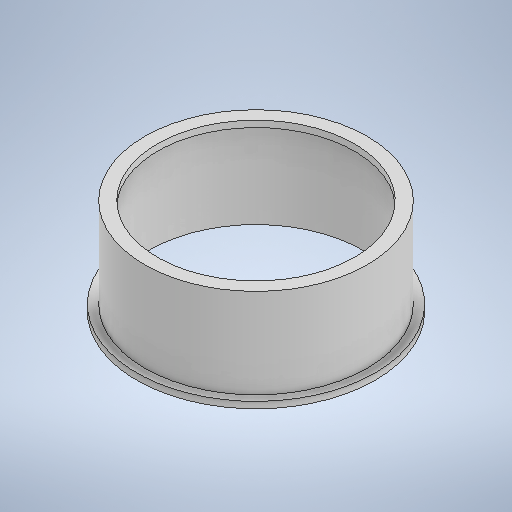
# Autodesk Inventor part: Cylinder Replacement- 10
Saved by Autodesk Inventor 2025.2 (Build 292293000, 293)
## iProperties
Created: 2024-04-11
Part Number: Cylinder Replacement- 10
Material: Generic
Document SubType Name: Modeling
Designer: Thienan Hoang
Density: 1 g/cm^3
Appearance: Default
Author: Thienan Hoang
Autodesk Inventor part; units mm, degrees
ref_plane "YZ Plane" through (0, 0, 0) normal (1, 0, 0) x (0, 1, 0)
ref_plane "XZ Plane" through (0, 0, 0) normal (0, 1, 0) x (-1, 0, 0)
sketch "Sketch1" plane through (0, 0, 0) normal (0, 1, 0) x (-1, 0, 0)
  circle A0 centre (0, 0) radius 74.5
  circle A1 centre (0, 0) radius 69.5
  circle A2 centre (0, 0) radius 66.5
  dimension "Absolute_Diameter" = 149
  dimension "Diameter_No_Outer_Lip" = 139
  dimension "Inner_Cylinder_Diameter" = 133
  constraints: 3 centre point, 3 coincident
  measures "Absolute_Diameter" diameter of A0
  measures "Diameter_No_Outer_Lip" diameter of A1
  measures "Inner_Cylinder_Diameter" diameter of A2
extrude "Extrusion1" add sketch "Sketch1" along normal blind 4 contours A0
extrude "Extrusion2" add sketch "Sketch1" along normal blind 60 contours A1
sketch "Sketch2" plane through (0, 60, 0) normal (0, 1, 0) x (1, 0, 0)
  circle A0 centre (0, 0) radius 61.5
  circle A1 centre (0, 0) radius 66.5
  dimension "Lip_Diameter_Out" = 123
  dimension "Top_Outer_Lip_Diameter" = 133
  constraints: 2 centre point, 2 coincident
  measures "Lip_Diameter_Out" diameter of A0
  measures "Top_Outer_Lip_Diameter" diameter of A1
extrude "Extrusion7" add sketch "Sketch2" against normal blind 4
ref_plane "Work Plane2" through (0, 10, 0) normal (0, 1, 0) x (1, 0, 0)
sketch "Sketch3" plane through (0, 10, 0) normal (0, 1, 0) x (1, 0, 0)
  circle A0 centre (0, 0) radius 127.5
  circle A1 centre (-127.5, 0) radius 2.5
  circle A2 centre (-103.1497, -74.9426) radius 2.5
  circle A3 centre (-39.3997, -121.2597) radius 2.5
  circle A4 centre (39.3997, -121.2597) radius 2.5
  circle A5 centre (103.1497, -74.9426) radius 2.5
  circle A6 centre (127.5, 0) radius 2.5
  circle A7 centre (103.1497, 74.9426) radius 2.5
  circle A8 centre (39.3997, 121.2597) radius 2.5
  circle A9 centre (-39.3997, 121.2597) radius 2.5
  circle A10 centre (-103.1497, 74.9426) radius 2.5
  dimension "d27" = 255
  dimension "d28" = 5
  dimension "d31" = 360
  constraints: 10 centre point, 1 coincident, 1 horizontal alignment, 23 other
  measures "d28" diameter of A1
extrude "Extrusion8" [suppressed]
sketch "Sketch24" plane through (0, 60, 0) normal (0, 1, 0) x (1, 0, 0)
  circle A0 centre (0, 0) radius 51
  circle A1 centre (0, -51) radius 2.75
  circle A2 centre (44.1673, -25.5) radius 2.75
  circle A3 centre (44.1673, 25.5) radius 2.75
  circle A4 centre (0, 51) radius 2.75
  circle A5 centre (-44.1673, 25.5) radius 2.75
  circle A6 centre (-44.1673, -25.5) radius 2.75
  dimension "d230" = 102
  dimension "d231" = 5.5
  dimension "d234" = 360
  constraints: 6 centre point, 1 coincident, 1 vertical alignment, 15 other
  measures "d231" diameter of A1
extrude "Extrusion30" [suppressed]
sketch "Sketch25" plane through (0, 60, 0) normal (0, 1, 0) x (1, 0, 0)
  point P0 (0, 0)
sketch "Sketch26" plane through (0, 60, 0) normal (0, 1, 0) x (1, 0, 0)
  circle A0 centre (-44.1673, 25.5) radius 2.75 projected
  circle A1 centre (0, 0) radius 51
  circle A2 centre (-51, 0) radius 3.25
  circle A3 centre (-25.5, -44.1673) radius 3.25
  circle A4 centre (25.5, -44.1673) radius 3.25
  circle A5 centre (51, 0) radius 3.25
  circle A6 centre (25.5, 44.1673) radius 3.25
  circle A7 centre (-25.5, 44.1673) radius 3.25
  dimension "d239" = 6.5
  dimension "d242" = 360
  constraints: 7 centre point, 2 point on circle, 1 coincident, 13 other
  measures "d239" diameter of A2
extrude "Extrusion31" [suppressed]
body "Solid1"
